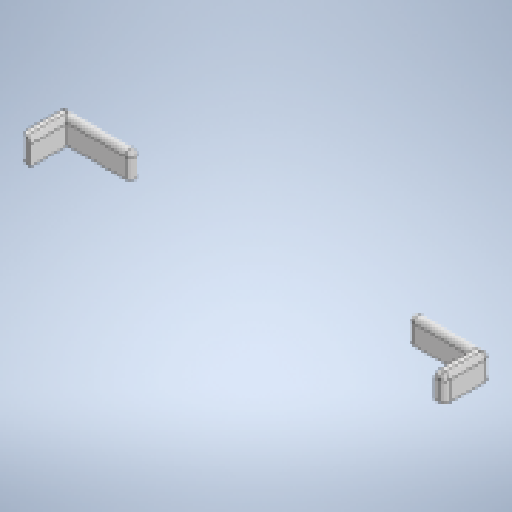
# Autodesk Inventor part: whiteboard-holder
Saved by Autodesk Inventor 2023 (Build 270158000, 158)
## iProperties
Created: 2022-10-03
Part Number: whiteboard-holder
Material: Generic
Document SubType Name: Modeling
Designer: carso
Density: 1 g/cm^3
Appearance: Default
Author: carso
Autodesk Inventor part; units mm, degrees
ref_plane "YZ Plane" through (0, 0, 0) normal (1, 0, 0) x (0, 1, 0)
ref_plane "XZ Plane" through (0, 0, 0) normal (0, 1, 0) x (-1, 0, 0)
ref_plane "XY Plane" through (0, 0, 0) normal (0, 0, 1) x (1, 0, 0)
sketch "Sketch1" plane through (0, 0, 0) normal (0, 1, 0) x (-1, 0, 0)
  line L0 (-8.8522, -15.6087) -> (166.1478, -15.6087)
  line L1 (166.1478, -15.6087) -> (166.1478, -19.6087)
  line L2 (166.1478, -19.6087) -> (-8.8522, -19.6087)
  line L3 (-8.8522, -19.6087) -> (-8.8522, -15.6087)
  line L4 (-8.8522, -15.6087) -> (-4.8522, -15.6087)
  line L5 (-4.8522, -15.6087) -> (-4.8522, -0.6087)
  line L6 (-4.8522, -0.6087) -> (-8.8522, -0.6087)
  line L7 (-8.8522, -0.6087) -> (-8.8522, -15.6087)
  line L8 (166.1478, -15.6087) -> (162.1478, -15.6087)
  line L9 (162.1478, -15.6087) -> (162.1478, -0.6087)
  line L10 (162.1478, -0.6087) -> (166.1478, -0.6087)
  line L11 (166.1478, -0.6087) -> (166.1478, -15.6087)
  line L12 (21.1478, -15.6087) -> (21.1478, -19.6087)
  line L13 (136.1478, -15.6087) -> (136.1478, -19.6087)
  point P0 (0, 0)
  point P1 (166.1478, -17.6087)
  point P2 (-8.8522, -17.6087)
  dimension "d2" = 4
  dimension "d3" = 4
  dimension "d4" = 175
  dimension "d5" = 15
  dimension "d7" = 4
  dimension "d8" = 15
  dimension "d9" = 30
  dimension "d10" = 30
  constraints: 28 end point, 6 parallel, 5 perpendicular, 4 point on line, 3 horizontal, 2 midpoint
  measures "d2" distance of L5.end L6.end
  measures "d3" distance between parallel lines of L2 L0
  measures "d4" distance of L1.end L2.end
  measures "d5" distance of L6.end L0.start
  measures "d7" distance of L9.end L10.end
  measures "d8" distance of L8.end L9.end
  measures "d9" distance from line of point (166.148, -17.609) L13
  measures "d10" distance from line of point (-8.852, -17.609) L12
extrude "Extrusion1" add sketch "Sketch1" along normal blind 10 contours L7 L6 L5 L0 | L0 L12 L2 L3 | L0 L1 L2 L13 | L9 L10 L11 L0
fillet "Fillet1" radius 2 10 edges at (-149.1478, 10, -15.6087) (-8.1478, 10, -15.6087) (8.8522, 10, -10.1087) (-6.1478, 10, -19.6087) (-151.1478, 10, -19.6087) (-166.1478, 5, -19.6087) (8.8522, 5, -19.6087) (8.8522, 5, -0.6087) (6.8522, 10, -0.6087) (-162.1478, 10, -8.1087)
fillet "Fillet2" radius 2 11 edges at (-21.1478, 4, -15.6087) (-21.1478, 4, -19.6087) (-21.1478, 9.4142, -19.0229) (-21.1478, 10, -17.6087) (-21.1478, 9.4142, -16.1945) (-136.1478, 4, -19.6087) (-136.1478, 4, -15.6087) (-136.1478, 10, -17.6087) (-136.1478, 9.4142, -16.1945) (-136.1478, 9.4142, -19.0229) (-166.1478, 5, -0.6087)
body "Solid1"
